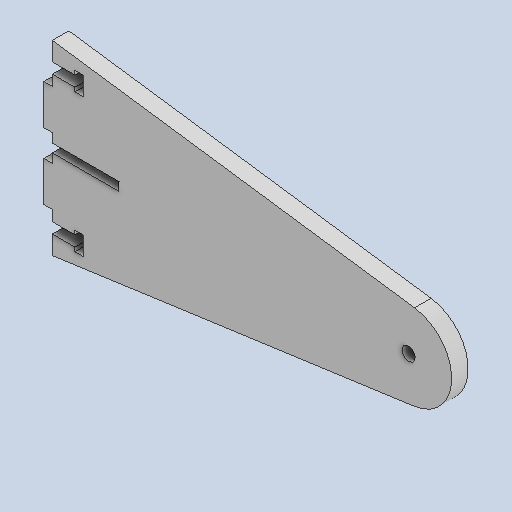
# Autodesk Inventor part: Base
Saved by Autodesk Inventor 2022 (Build 260153000, 153)
## iProperties
Created: 2022-02-08
Part Number: Base
Material: Generic
Document SubType Name: Modeling
Designer: katha
Density: 1 g/cm^3
Appearance: Default
Author: katha
Autodesk Inventor part; units mm, degrees
ref_plane "YZ Plane" through (0, 0, 0) normal (1, 0, 0) x (0, 1, 0)
ref_plane "XZ Plane" through (0, 0, 0) normal (0, 1, 0) x (-1, 0, 0)
ref_plane "XY Plane" through (0, 0, 0) normal (0, 0, 1) x (1, 0, 0)
sketch "Sketch2" plane through (0, 0, 0) normal (0, 0, 1) x (1, 0, 0)
  arc A0 (9.9386, -9.7664) -> (20.0614, -9.7664) centre (15, 0) ccw
  arc A1 (20.9272, -9.2665) -> (25.9886, -0.4999) centre (15, 0) ccw
  arc A2 (25.9886, 0.4999) -> (20.9272, 9.2665) centre (15, 0) ccw
  arc A3 (20.0614, 9.7664) -> (9.9386, 9.7664) centre (15, 0) ccw
  arc A4 (9.0728, 9.2665) -> (4.0114, 0.4999) centre (15, 0) ccw
  arc A5 (4.0114, -0.4999) -> (9.0728, -9.2665) centre (15, 0) ccw
  circle A6 centre (15, 0) radius 2.5
  arc A7 (0, -3) -> (12, -15) centre (12, -3) ccw
  circle A8 centre (15, 0) radius 16.1883
  line L0 (31.1883, 0) -> (-118.8117, 0) construction
  line L1 (-118.8117, 0) -> (-118.8117, 35)
  line L2 (17.2352, 16.0332) -> (-118.8117, 35)
  line L3 (-118.8117, 0) -> (-118.8117, -35)
  line L4 (17.2352, -16.0332) -> (-118.8117, -35)
  line L5 (-118.8117, -20) -> (-122.0117, -20)
  line L6 (-122.0117, -20) -> (-122.0117, -5)
  line L7 (-122.0117, -5) -> (-118.8117, -5)
  line L8 (-118.8117, 20) -> (-122.0117, 20)
  line L9 (-122.0117, 20) -> (-122.0117, 5)
  line L10 (-122.0117, 5) -> (-118.8117, 5)
  line L11 (-118.8117, 0) -> (-118.8117, 1.6)
  line L12 (-118.8117, 1.6) -> (-93.8117, 1.6)
  line L13 (-118.8117, 0) -> (-118.8117, -1.6)
  line L14 (-118.8117, -1.6) -> (-93.8117, -1.6)
  line L15 (-93.8117, -1.6) -> (-93.8117, 1.6)
  point P0 (0, 0)
  point P1 (5.2336, -12.9104)
  point P2 (2.0896, -9.7664)
  point P3 (-118.8117, 5)
  point P4 (-118.8117, 20)
extrude "Extrusion1" add sketch "Sketch2" along normal blind 6.2
sketch "Sketch4" plane through (0, 0, 0) normal (0, 0, -1) x (-1, 0, 0)
  line L0 (93.8117, -1.6) -> (93.8117, 1.6) projected
  line L1 (118.8117, 1.6) -> (93.8117, 1.6) projected
  line L2 (118.8117, -1.6) -> (93.8117, -1.6) projected
  line L3 (118.8117, 5) -> (118.8117, -5) projected
  line L4 (118.8117, 0) -> (118.8117, -35) projected
  point P0 (0, 0)
extrude "Extrusion2" cut sketch "Sketch4" against normal blind 10
sketch "Sketch5" plane through (0, 0, 0) normal (0, 0, -1) x (-1, 0, 0)
  line L0 (118.8117, -111.6) -> (118.8117, 288.4) projected
  line L1 (118.8117, -20) -> (118.8117, -35) projected
  line L2 (118.8117, -24) -> (110.3117, -24)
  line L3 (110.3117, -24) -> (110.3117, -28)
  line L4 (110.3117, -28) -> (118.8117, -28)
  line L5 (118.8117, -28) -> (118.8117, -24)
  line L6 (110.3117, -26) -> (110.3117, -22.5)
  line L7 (110.3117, -22.5) -> (107.1117, -22.5)
  line L8 (110.3117, -26) -> (112.3394, -26) construction
  line L9 (110.3117, -26) -> (110.3117, -29.5)
  line L10 (110.3117, -29.5) -> (107.1117, -29.5)
  line L11 (107.1117, -29.5) -> (107.1117, -22.5)
  line L12 (93.8117, -1.6) -> (93.8117, 1.6) projected
  line L13 (93.8117, 0) -> (107.5488, 0) construction
  line L14 (118.8117, 111.6) -> (118.8117, -288.4)
  line L15 (118.8117, 20) -> (118.8117, 35)
  line L16 (118.8117, 24) -> (110.3117, 24)
  line L17 (110.3117, 28) -> (118.8117, 28)
  line L18 (110.3117, 26) -> (110.3117, 22.5)
  line L19 (110.3117, 22.5) -> (107.1117, 22.5)
  line L20 (110.3117, 26) -> (110.3117, 29.5)
  line L21 (110.3117, 29.5) -> (107.1117, 29.5)
  line L22 (107.1117, 29.5) -> (107.1117, 22.5)
  point P0 (0, 0)
  dimension "d14" = 8.5
  dimension "d15" = 4
  dimension "d16" = 7
  dimension "d17" = 3.5
  dimension "d18" = 3.2
  constraints: 40 end point, 15 symmetric about line, 3 horizontal, 2 midpoint, 2 parallel, 2 perpendicular, 2 point on line, 2 vertical
  measures "d14" distance of L4.end L3.end
  measures "d15" distance of L3.end L2.end
  measures "d16" distance from line of L4 L1.end
  measures "d17" distance of L6.start L6.end
  measures "d18" distance of L6.end L7.end
extrude "Extrusion3" cut sketch "Sketch5" against normal blind 6.2
body "Solid1"
